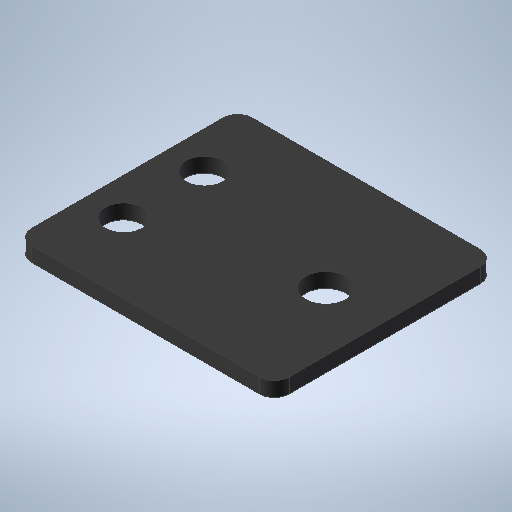
# Autodesk Inventor part: Part20
Saved by Autodesk Inventor 2025.2 (Build 292293000, 293)
## iProperties
Created: 2026-03-31
Part Number: Part20
Material: Generic
Document SubType Name: Modeling
Designer: composite
Density: 1 g/cm^3
Appearance: Default
Author: composite
Autodesk Inventor part; units mm, degrees
ref_plane "YZ Plane" through (0, 0, 0) normal (1, 0, 0) x (0, 1, 0)
ref_plane "XZ Plane" through (0, 0, 0) normal (0, 1, 0) x (-1, 0, 0)
ref_plane "XY Plane" through (0, 0, 0) normal (0, 0, 1) x (1, 0, 0)
sketch "Sketch1" plane through (0, 0, 0) normal (0, 1, 0) x (-1, 0, 0)
  line L0 (0, 0) -> (35, 0)
  line L1 (35, 0) -> (35, -30)
  line L2 (35, -30) -> (0, -30)
  line L3 (0, -30) -> (0, 0)
  circle A0 centre (30, -9.5) radius 2.5
  circle A1 centre (30, -20.5) radius 2.5
  line L4 (30, -9.5) -> (30, -20.5) construction
  circle A2 centre (8, -15) radius 2.75
  point P0 (35, -15)
  point P1 (30, -15)
  point P2 (0, -15)
  dimension "d0" = 30
  dimension "d1" = 35
  dimension "d2" = 5
  dimension "d3" = 5
  dimension "d4" = 11
  dimension "d5" = 5
  dimension "d6" = 5.5
  dimension "d7" = 8
  constraints: 10 end point, 3 centre point, 3 midpoint, 2 horizontal alignment, 2 parallel, 1 horizontal, 1 perpendicular, 1 vertical, 1 vertical alignment
  measures "d0" distance of L0.end L1.end
  measures "d1" distance of L1.end L2.end
  measures "d2" diameter of A0
  measures "d3" diameter of A1
  measures "d4" distance of L4.end L4.start
  measures "d5" distance from line of L1 L4.start
  measures "d6" diameter of A2
  measures "d7" distance from line of L3 A2.centre
extrude "Extrusion1" add sketch "Sketch1" along normal blind 2
fillet "Fillet1" radius 2 4 edges at (0, 1, -30) (0, 1, 0) (-35, 1, 0) (-35, 1, -30)
equation "\"d3\" = d2"
body "Solid1"
